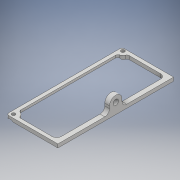
# Autodesk Inventor part: bousetrapHolder
Saved by Autodesk Inventor 2018.3 (Build 223284000, 284)
## iProperties
Created: 2018-06-30
Part Number: bousetrapHolder
Material: Generic
Document SubType Name: Modeling
Designer: mzhang
Density: 1 g/cm^3
Appearance: Default
Author: mzhang
Autodesk Inventor part; units mm, degrees
ref_plane "YZ Plane" through (0, 0, 0) normal (1, 0, 0) x (0, 1, 0)
ref_plane "XZ Plane" through (0, 0, 0) normal (0, 1, 0) x (-1, 0, 0)
ref_plane "XY Plane" through (0, 0, 0) normal (0, 0, 1) x (1, 0, 0)
sketch "Sketch1" plane through (0, 0, 0) normal (0, 0, 1) x (1, 0, 0)
  line L0 (0, 0) -> (43.5, 0)
  line L1 (43.5, 97.7504) -> (0, 97.7504)
  line L2 (0, 97.7504) -> (0, 0)
  line L3 (7.4492, 94.7504) -> (39.5, 94.7504)
  line L4 (39.5, 3) -> (7.5, 3)
  line L5 (3, 7.5) -> (3, 90.925)
  circle A0 centre (3, 95.425) radius 1.5
  circle A1 centre (3, 3) radius 1.5
  arc A2 (7.5, 3) -> (3, 7.5) centre (3, 3) ccw
  arc A3 (3, 90.925) -> (7.4492, 94.7504) centre (3, 95.425) ccw
  line L6 (43.5, 94.7504) -> (43.5, 0)
  line L7 (39.5, 3) -> (39.5, 94.7504)
  line L8 (43.5, 97.7504) -> (43.5, 94.7504)
  dimension "d3" = 3
  dimension "d4" = 3
  dimension "d5" = 3
  dimension "d8" = 3
  dimension "d11" = 3
  dimension "d31" = 39.5
  dimension "d32" = 43.5
  constraints: 18 end point, 4 centre point, 4 point on circle, 3 parallel, 1 horizontal, 1 vertical
  measures "d3" distance between parallel lines of L1 L3
  measures "d4" diameter of A0
  measures "d5" diameter of A1
  measures "d8" radial gap between concentric circles of A1 A2
  measures "d11" radial gap between concentric circles of A0 A3
  measures "d31" distance between parallel lines of L7 L2
  measures "d32" distance between parallel lines of L6 L2
extrude "Extrusion1" add sketch "Sketch1" along normal blind 3
fillet "Fillet1" radius 2 2 edges at (0, 97.7504, 1.5) (0, 0, 1.5)
fillet "Fillet2" radius 4 2 edges at (39.5, 94.7504, 1.5) (39.5, 3, 1.5)
fillet "Fillet3" radius 2 4 edges at (7.4492, 94.7504, 1.5) (3, 90.925, 1.5) (3, 7.5, 1.5) (7.5, 3, 1.5)
sketch "Sketch2" plane through (43.5, 2, 0) normal (1, 0, 0) x (0, 0, -1)
  circle A0 centre (-9, 46.8752) radius 2.25
  circle A1 centre (-9, 46.8752) radius 5.25
  line L0 (-9, 41.6252) -> (-3, 41.6252)
  line L1 (0, 5) -> (0, 88.7504) projected
  line L2 (-9, 52.1252) -> (-3, 52.1252)
  line L3 (0, -2) -> (0, 95.7504) projected
  line L4 (-3, -2) -> (-3, 95.7504) projected
  line L5 (0, -2) -> (0, 95.7504) projected
  line L6 (0, 95.7504) -> (-3, 95.7504) projected
  line L7 (0, -2) -> (-3, -2) projected
  point P0 (0, 0)
  point P1 (0, 93.7504)
  dimension "d21" = 4.5
  dimension "d22" = 3
  dimension "d23" = 9
  constraints: 4 end point, 2 centre point, 2 point on circle, 2 point on line, 1 horizontal, 1 perpendicular, 1 other
  measures "d21" diameter of A0
  measures "d22" radial gap between concentric circles of A0 A1
  measures "d23" distance from line of L1 A0.centre
extrude "Extrusion2" add sketch "Sketch2" against normal up to surface (4 mm away) contours A1 | A1 L2 L4 L0
fillet "Fillet4" radius 4 2 edges at (41.5, 43.6252, 3) (41.5, 54.1252, 3)
sketch "Sketch3" plane through (2, 0, 0) normal (0, -1, 0) x (1, 0, 0)
  line L0 (-0.5, 3) -> (2.5, 3) projected
  circle A0 centre (1, -3) radius 4
  line L1 (0, 3) -> (41.5, 3) projected
  point P0 (-2, 0)
  point P1 (1, 3)
  point P2 (42, 3)
  dimension "d27" = 8
  dimension "d28" = 6
  constraints: 1 centre point, 1 midpoint
  measures "d27" diameter of A0
  measures "d28" distance from line of A0.centre L1
extrude "Extrusion3" cut sketch "Sketch3" against normal up to surface (97.7504 mm away)
body "Solid1"
